Autodesk Inventor part; units mm, degrees
(part 2 of 6)
  line L607 (-11.5427, -57.3701) -> (-11.3963, -57.3701) construction
  spline S77 degree 2 poles (-11.3963, -57.3701) (-11.2792, -57.3701) (-11.0841, -57.5457) (-11.0841, -57.6677) knots 0 0 0 1 2 2 2
  line L608 (-11.3963, -57.3701) -> (-11.2792, -57.3701) construction
  line L609 (-11.2792, -57.3701) -> (-11.0841, -57.5457) construction
  line L610 (-11.0841, -57.5457) -> (-11.0841, -57.6677) construction
  spline S78 degree 2 poles (-11.0841, -57.6677) (-11.0841, -57.7506) (-11.1378, -57.8336) knots 0 0 0 1 1 1
  line L611 (-11.0841, -57.6677) -> (-11.0841, -57.7506) construction
  line L612 (-11.0841, -57.7506) -> (-11.1378, -57.8336) construction
  spline S79 degree 2 poles (-11.1378, -61.0047) (-11.0841, -61.0876) (-11.0841, -61.1705) knots 0 0 0 1 1 1
  line L613 (-11.1378, -61.0047) -> (-11.0841, -61.0876) construction
  line L614 (-11.0841, -61.0876) -> (-11.0841, -61.1705) construction
  spline S80 degree 2 poles (-11.0841, -61.1705) (-11.0841, -61.2925) (-11.2792, -61.4681) (-11.3963, -61.4681) knots 0 0 0 1 2 2 2
  line L615 (-11.0841, -61.1705) -> (-11.0841, -61.2925) construction
  line L616 (-11.0841, -61.2925) -> (-11.2792, -61.4681) construction
  line L617 (-11.2792, -61.4681) -> (-11.3963, -61.4681) construction
  spline S81 degree 2 poles (-21.1899, -61.1305) (-21.2987, -61.4569) (-21.5482, -61.4569) knots 0 0 0 1 1 1
  line L618 (-21.1899, -61.1305) -> (-21.2987, -61.4569) construction
  line L619 (-21.2987, -61.4569) -> (-21.5482, -61.4569) construction
  spline S82 degree 2 poles (-21.5482, -61.4569) (-21.8041, -61.4569) (-21.9065, -61.1305) knots 0 0 0 1 1 1
  line L620 (-21.5482, -61.4569) -> (-21.8041, -61.4569) construction
  line L621 (-21.8041, -61.4569) -> (-21.9065, -61.1305) construction
  line L622 (-21.9065, -61.1305) -> (-24.2098, -54.3101)
  spline S83 degree 2 poles (-24.2098, -54.3101) (-24.229, -54.2397) (-24.229, -54.1693) knots 0 0 0 1 1 1
  line L623 (-24.2098, -54.3101) -> (-24.229, -54.2397) construction
  line L624 (-24.229, -54.2397) -> (-24.229, -54.1693) construction
  spline S84 degree 2 poles (-24.229, -54.1693) (-24.229, -53.8046) (-23.8323, -53.8046) knots 0 0 0 1 1 1
  line L625 (-24.229, -54.1693) -> (-24.229, -53.8046) construction
  line L626 (-24.229, -53.8046) -> (-23.8323, -53.8046) construction
  spline S85 degree 2 poles (-23.8323, -53.8046) (-23.5764, -53.8046) (-23.4868, -54.0669) knots 0 0 0 1 1 1
  line L627 (-23.8323, -53.8046) -> (-23.5764, -53.8046) construction
  line L628 (-23.5764, -53.8046) -> (-23.4868, -54.0669) construction
  spline S86 degree 2 poles (-19.6095, -54.0669) (-19.52, -53.8046) (-19.264, -53.8046) knots 0 0 0 1 1 1
  line L629 (-19.6095, -54.0669) -> (-19.52, -53.8046) construction
  line L630 (-19.52, -53.8046) -> (-19.264, -53.8046) construction
  spline S87 degree 2 poles (-19.264, -53.8046) (-18.8673, -53.8046) (-18.8673, -54.1693) knots 0 0 0 1 1 1
  line L631 (-19.264, -53.8046) -> (-18.8673, -53.8046) construction
  line L632 (-18.8673, -53.8046) -> (-18.8673, -54.1693) construction
  spline S88 degree 2 poles (-18.8673, -54.1693) (-18.8673, -54.2397) (-18.8929, -54.3101) knots 0 0 0 1 1 1
  line L633 (-18.8673, -54.1693) -> (-18.8673, -54.2397) construction
  line L634 (-18.8673, -54.2397) -> (-18.8929, -54.3101) construction
  line L635 (-18.8929, -54.3101) -> (-21.1899, -61.1305)
  spline S89 degree 2 poles (16.563, -43.9283) (16.3391, -43.9283) (16.0871, -44.2083) (16.0871, -44.4042) knots 0 0 0 1 2 2 2
  line L636 (16.563, -43.9283) -> (16.3391, -43.9283) construction
  line L637 (16.3391, -43.9283) -> (16.0871, -44.2083) construction
  line L638 (16.0871, -44.2083) -> (16.0871, -44.4042) construction
  spline S90 degree 2 poles (16.0871, -44.4042) (16.0871, -44.6002) (16.2071, -44.7361) knots 0 0 0 1 1 1
  line L639 (16.0871, -44.4042) -> (16.0871, -44.6002) construction
  line L640 (16.0871, -44.6002) -> (16.2071, -44.7361) construction
  spline S91 degree 2 poles (16.2071, -44.7361) (16.3391, -44.8841) (16.563, -44.8841) knots 0 0 0 1 1 1
  line L641 (16.2071, -44.7361) -> (16.3391, -44.8841) construction
  line L642 (16.3391, -44.8841) -> (16.563, -44.8841) construction
  spline S92 degree 2 poles (16.0471, -46.6916) (15.9752, -46.8035) (15.8552, -46.8035) knots 0 0 0 1 1 1
  line L643 (16.0471, -46.6916) -> (15.9752, -46.8035) construction
  line L644 (15.9752, -46.8035) -> (15.8552, -46.8035) construction
  spline S93 degree 2 poles (15.8552, -46.8035) (15.7552, -46.8035) (15.6033, -46.6596) (15.6033, -46.5636) knots 0 0 0 1 2 2 2
  line L645 (15.8552, -46.8035) -> (15.7552, -46.8035) construction
  line L646 (15.7552, -46.8035) -> (15.6033, -46.6596) construction
  line L647 (15.6033, -46.6596) -> (15.6033, -46.5636) construction
  spline S94 degree 2 poles (15.6033, -46.5636) (15.6033, -46.4916) (15.6473, -46.4276) knots 0 0 0 1 1 1
  line L648 (15.6033, -46.5636) -> (15.6033, -46.4916) construction
  line L649 (15.6033, -46.4916) -> (15.6473, -46.4276) construction
  line L650 (15.6473, -46.4276) -> (16.3671, -45.3479)
  spline S95 degree 2 poles (16.3671, -45.3479) (16.0072, -45.288) (15.7952, -45.004) knots 0 0 0 1 1 1
  line L651 (16.3671, -45.3479) -> (16.0072, -45.288) construction
  line L652 (16.0072, -45.288) -> (15.7952, -45.004) construction
  spline S96 degree 2 poles (15.7952, -45.004) (15.6073, -44.7481) (15.6073, -44.4042) knots 0 0 0 1 1 1
  line L653 (15.7952, -45.004) -> (15.6073, -44.7481) construction
  line L654 (15.6073, -44.7481) -> (15.6073, -44.4042) construction
  spline S97 degree 2 poles (15.6073, -44.4042) (15.6073, -44.0163) (15.8472, -43.7484) knots 0 0 0 1 1 1
  line L655 (15.6073, -44.4042) -> (15.6073, -44.0163) construction
  line L656 (15.6073, -44.0163) -> (15.8472, -43.7484) construction
  spline S98 degree 2 poles (15.8472, -43.7484) (16.1111, -43.4485) (16.563, -43.4485) knots 0 0 0 1 1 1
  line L657 (15.8472, -43.7484) -> (16.1111, -43.4485) construction
  line L658 (16.1111, -43.4485) -> (16.563, -43.4485) construction
  line L659 (16.563, -43.4485) -> (17.7587, -43.4485)
  spline S99 degree 2 poles (17.7587, -43.4485) (17.9986, -43.4485) (17.9986, -43.6884) knots 0 0 0 1 1 1
  line L660 (17.7587, -43.4485) -> (17.9986, -43.4485) construction
  line L661 (17.9986, -43.4485) -> (17.9986, -43.6884) construction
  line L662 (17.9986, -43.6884) -> (17.9986, -46.5596)
  spline S100 degree 2 poles (17.9986, -46.5596) (17.9986, -46.7995) (17.7587, -46.7995) knots 0 0 0 1 1 1
  line L663 (17.9986, -46.5596) -> (17.9986, -46.7995) construction
  line L664 (17.9986, -46.7995) -> (17.7587, -46.7995) construction
  spline S101 degree 2 poles (17.7587, -46.7995) (17.5187, -46.7995) (17.5187, -46.5596) knots 0 0 0 1 1 1
  line L665 (17.7587, -46.7995) -> (17.5187, -46.7995) construction
  line L666 (17.5187, -46.7995) -> (17.5187, -46.5596) construction
  spline S102 degree 2 poles (13.6918, -46.3197) (13.8878, -46.3197) (14.1677, -46.0357) (14.1677, -45.8398) knots 0 0 0 1 2 2 2
  line L667 (13.6918, -46.3197) -> (13.8878, -46.3197) construction
  line L668 (13.8878, -46.3197) -> (14.1677, -46.0357) construction
  line L669 (14.1677, -46.0357) -> (14.1677, -45.8398) construction
  spline S103 degree 2 poles (13.2119, -43.9283) (13.016, -43.9283) (12.7361, -44.2123) (12.7361, -44.4082) knots 0 0 0 1 2 2 2
  line L670 (13.2119, -43.9283) -> (13.016, -43.9283) construction
  line L671 (13.016, -43.9283) -> (12.7361, -44.2123) construction
  line L672 (12.7361, -44.2123) -> (12.7361, -44.4082) construction
  line L673 (12.7361, -44.4082) -> (12.7361, -45.8398)
  spline S104 degree 2 poles (12.7361, -45.8398) (12.7361, -46.0357) (13.016, -46.3197) (13.2119, -46.3197) knots 0 0 0 1 2 2 2
  line L674 (12.7361, -45.8398) -> (12.7361, -46.0357) construction
  line L675 (12.7361, -46.0357) -> (13.016, -46.3197) construction
  line L676 (13.016, -46.3197) -> (13.2119, -46.3197) construction
  line L677 (13.2119, -46.3197) -> (13.6918, -46.3197)
  line L678 (13.6918, -46.7995) -> (13.2119, -46.7995)
  spline S105 degree 2 poles (13.2119, -46.7995) (12.8201, -46.7995) (12.2562, -46.2397) (12.2562, -45.8438) knots 0 0 0 1 2 2 2
  line L679 (13.2119, -46.7995) -> (12.8201, -46.7995) construction
  line L680 (12.8201, -46.7995) -> (12.2562, -46.2397) construction
  line L681 (12.2562, -46.2397) -> (12.2562, -45.8438) construction
  line L682 (12.2562, -45.8438) -> (12.2562, -44.4042)
  spline S106 degree 2 poles (12.2562, -44.4042) (12.2562, -44.0083) (12.8201, -43.4485) (13.2119, -43.4485) knots 0 0 0 1 2 2 2
  line L683 (12.2562, -44.4042) -> (12.2562, -44.0083) construction
  line L684 (12.2562, -44.0083) -> (12.8201, -43.4485) construction
  line L685 (12.8201, -43.4485) -> (13.2119, -43.4485) construction
  line L686 (13.2119, -43.4485) -> (14.4076, -43.4485)
  spline S107 degree 2 poles (14.4076, -43.4485) (14.6475, -43.4485) (14.6475, -43.6884) knots 0 0 0 1 1 1
  line L687 (14.4076, -43.4485) -> (14.6475, -43.4485) construction
  line L688 (14.6475, -43.4485) -> (14.6475, -43.6884) construction
  line L689 (14.6475, -43.6884) -> (14.6475, -45.8358)
  spline S108 degree 2 poles (14.6475, -45.8358) (14.6475, -46.1957) (14.9834, -46.3397) knots 0 0 0 1 1 1
  line L690 (14.6475, -45.8358) -> (14.6475, -46.1957) construction
  line L691 (14.6475, -46.1957) -> (14.9834, -46.3397) construction
  spline S109 degree 2 poles (14.9834, -46.3397) (15.1314, -46.3996) (15.1314, -46.5516) knots 0 0 0 1 1 1
  line L692 (14.9834, -46.3397) -> (15.1314, -46.3996) construction
  line L693 (15.1314, -46.3996) -> (15.1314, -46.5516) construction
  spline S110 degree 2 poles (15.1314, -46.5516) (15.1314, -46.6516) (14.9954, -46.8035) (14.8955, -46.8035) knots 0 0 0 1 2 2 2
  line L694 (15.1314, -46.5516) -> (15.1314, -46.6516) construction
  line L695 (15.1314, -46.6516) -> (14.9954, -46.8035) construction
  line L696 (14.9954, -46.8035) -> (14.8955, -46.8035) construction
  spline S111 degree 2 poles (14.8955, -46.8035) (14.8435, -46.8035) (14.7915, -46.7795) knots 0 0 0 1 1 1
  line L697 (14.8955, -46.8035) -> (14.8435, -46.8035) construction
  line L698 (14.8435, -46.8035) -> (14.7915, -46.7795) construction
  spline S112 degree 2 poles (14.7915, -46.7795) (14.5516, -46.6756) (14.4036, -46.4836) knots 0 0 0 1 1 1
  line L699 (14.7915, -46.7795) -> (14.5516, -46.6756) construction
  line L700 (14.5516, -46.6756) -> (14.4036, -46.4836) construction
  spline S113 degree 2 poles (14.4036, -46.4836) (14.1157, -46.7995) (13.6918, -46.7995) knots 0 0 0 1 1 1
  line L701 (14.4036, -46.4836) -> (14.1157, -46.7995) construction
  line L702 (14.1157, -46.7995) -> (13.6918, -46.7995) construction
  spline S114 degree 2 poles (-0.9121, -46.7995) (-1.152, -46.7995) (-1.152, -46.5596) knots 0 0 0 1 1 1
  line L703 (-0.9121, -46.7995) -> (-1.152, -46.7995) construction
  line L704 (-1.152, -46.7995) -> (-1.152, -46.5596) construction
  spline S115 degree 2 poles (-2.5996, -46.6356) (-2.6516, -46.7995) (-2.8115, -46.7995) knots 0 0 0 1 1 1
  line L705 (-2.5996, -46.6356) -> (-2.6516, -46.7995) construction
  line L706 (-2.6516, -46.7995) -> (-2.8115, -46.7995) construction
  spline S116 degree 2 poles (-2.8115, -46.7995) (-3.0635, -46.7995) (-3.0635, -46.5716) knots 0 0 0 1 1 1
  line L707 (-2.8115, -46.7995) -> (-3.0635, -46.7995) construction
  line L708 (-3.0635, -46.7995) -> (-3.0635, -46.5716) construction
  spline S117 degree 2 poles (-3.0635, -46.5716) (-3.0635, -46.5276) (-3.0475, -46.4836) knots 0 0 0 1 1 1
  line L709 (-3.0635, -46.5716) -> (-3.0635, -46.5276) construction
  line L710 (-3.0635, -46.5276) -> (-3.0475, -46.4836) construction
  line L711 (-3.0475, -46.4836) -> (-2.0997, -43.6124)
  spline S118 degree 2 poles (-2.0997, -43.6124) (-2.0478, -43.4485) (-1.8758, -43.4485) knots 0 0 0 1 1 1
  line L712 (-2.0997, -43.6124) -> (-2.0478, -43.4485) construction
  line L713 (-2.0478, -43.4485) -> (-1.8758, -43.4485) construction
  line L714 (-1.8758, -43.4485) -> (-0.9121, -43.4485)
  spline S119 degree 2 poles (-0.9121, -43.4485) (-0.6721, -43.4485) (-0.6721, -43.6884) knots 0 0 0 1 1 1
  line L715 (-0.9121, -43.4485) -> (-0.6721, -43.4485) construction
  line L716 (-0.6721, -43.4485) -> (-0.6721, -43.6884) construction
  line L717 (-0.6721, -43.6884) -> (-0.6721, -46.5596)
  spline S120 degree 2 poles (-0.6721, -46.5596) (-0.6721, -46.7995) (-0.9121, -46.7995) knots 0 0 0 1 1 1
  line L718 (-0.6721, -46.5596) -> (-0.6721, -46.7995) construction
  line L719 (-0.6721, -46.7995) -> (-0.9121, -46.7995) construction
  spline S121 degree 2 poles (-14.3163, -46.7995) (-14.5562, -46.7995) (-14.5562, -46.5596) knots 0 0 0 1 1 1
  line L720 (-14.3163, -46.7995) -> (-14.5562, -46.7995) construction
  line L721 (-14.5562, -46.7995) -> (-14.5562, -46.5596) construction
  line L722 (-14.5562, -46.5596) -> (-14.5562, -44.4082)
  spline S122 degree 2 poles (-14.5562, -44.4082) (-14.5562, -44.2123) (-14.8362, -43.9283) (-15.0321, -43.9283) knots 0 0 0 1 2 2 2
  line L723 (-14.5562, -44.4082) -> (-14.5562, -44.2123) construction
  line L724 (-14.5562, -44.2123) -> (-14.8362, -43.9283) construction
  line L725 (-14.8362, -43.9283) -> (-15.0321, -43.9283) construction
  spline S123 degree 2 poles (-15.9878, -46.5596) (-15.9878, -46.7995) (-16.2278, -46.7995) knots 0 0 0 1 1 1
  line L726 (-15.9878, -46.5596) -> (-15.9878, -46.7995) construction
  line L727 (-15.9878, -46.7995) -> (-16.2278, -46.7995) construction
  spline S124 degree 2 poles (-16.2278, -46.7995) (-16.4677, -46.7995) (-16.4677, -46.5596) knots 0 0 0 1 1 1
  line L728 (-16.2278, -46.7995) -> (-16.4677, -46.7995) construction
  line L729 (-16.4677, -46.7995) -> (-16.4677, -46.5596) construction
  line L730 (-16.4677, -46.5596) -> (-16.4677, -43.6884)
  spline S125 degree 2 poles (-16.4677, -43.6884) (-16.4677, -43.4485) (-16.2278, -43.4485) knots 0 0 0 1 1 1
  line L731 (-16.4677, -43.6884) -> (-16.4677, -43.4485) construction
  line L732 (-16.4677, -43.4485) -> (-16.2278, -43.4485) construction
  line L733 (-16.2278, -43.4485) -> (-15.0321, -43.4485)
  spline S126 degree 2 poles (-15.0321, -43.4485) (-14.6362, -43.4485) (-14.0764, -44.0083) (-14.0764, -44.4042) knots 0 0 0 1 2 2 2
  line L734 (-15.0321, -43.4485) -> (-14.6362, -43.4485) construction
  line L735 (-14.6362, -43.4485) -> (-14.0764, -44.0083) construction
  line L736 (-14.0764, -44.0083) -> (-14.0764, -44.4042) construction
  line L737 (-14.0764, -44.4042) -> (-14.0764, -46.5596)
  spline S127 degree 2 poles (-14.0764, -46.5596) (-14.0764, -46.7995) (-14.3163, -46.7995) knots 0 0 0 1 1 1
  line L738 (-14.0764, -46.5596) -> (-14.0764, -46.7995) construction
  line L739 (-14.0764, -46.7995) -> (-14.3163, -46.7995) construction
  spline S128 degree 2 poles (-18.3832, -46.3197) (-18.1872, -46.3197) (-17.9073, -46.0357) (-17.9073, -45.8398) knots 0 0 0 1 2 2 2
  line L740 (-18.3832, -46.3197) -> (-18.1872, -46.3197) construction
  line L741 (-18.1872, -46.3197) -> (-17.9073, -46.0357) construction
  line L742 (-17.9073, -46.0357) -> (-17.9073, -45.8398) construction
  spline S129 degree 2 poles (-18.863, -43.9283) (-19.059, -43.9283) (-19.3389, -44.2123) (-19.3389, -44.4082) knots 0 0 0 1 2 2 2
  line L743 (-18.863, -43.9283) -> (-19.059, -43.9283) construction
  line L744 (-19.059, -43.9283) -> (-19.3389, -44.2123) construction
  line L745 (-19.3389, -44.2123) -> (-19.3389, -44.4082) construction
  line L746 (-19.3389, -44.4082) -> (-19.3389, -45.8398)
  spline S130 degree 2 poles (-19.3389, -45.8398) (-19.3389, -46.0357) (-19.059, -46.3197) (-18.863, -46.3197) knots 0 0 0 1 2 2 2
  line L747 (-19.3389, -45.8398) -> (-19.3389, -46.0357) construction
  line L748 (-19.3389, -46.0357) -> (-19.059, -46.3197) construction
  line L749 (-19.059, -46.3197) -> (-18.863, -46.3197) construction
  line L750 (-18.863, -46.3197) -> (-18.3832, -46.3197)
  line L751 (-18.3832, -46.7995) -> (-18.863, -46.7995)
  spline S131 degree 2 poles (-18.863, -46.7995) (-19.2549, -46.7995) (-19.8188, -46.2397) (-19.8188, -45.8438) knots 0 0 0 1 2 2 2
  line L752 (-18.863, -46.7995) -> (-19.2549, -46.7995) construction
  line L753 (-19.2549, -46.7995) -> (-19.8188, -46.2397) construction
  line L754 (-19.8188, -46.2397) -> (-19.8188, -45.8438) construction
  line L755 (-19.8188, -45.8438) -> (-19.8188, -44.4042)
  spline S132 degree 2 poles (-19.8188, -44.4042) (-19.8188, -44.0083) (-19.2549, -43.4485) (-18.863, -43.4485) knots 0 0 0 1 2 2 2
  line L756 (-19.8188, -44.4042) -> (-19.8188, -44.0083) construction
  line L757 (-19.8188, -44.0083) -> (-19.2549, -43.4485) construction
  line L758 (-19.2549, -43.4485) -> (-18.863, -43.4485) construction
  line L759 (-18.863, -43.4485) -> (-17.6674, -43.4485)
  spline S133 degree 2 poles (-17.6674, -43.4485) (-17.4274, -43.4485) (-17.4274, -43.6884) knots 0 0 0 1 1 1
  line L760 (-17.6674, -43.4485) -> (-17.4274, -43.4485) construction
  line L761 (-17.4274, -43.4485) -> (-17.4274, -43.6884) construction
  line L762 (-17.4274, -43.6884) -> (-17.4274, -45.8358)
  spline S134 degree 2 poles (-17.4274, -45.8358) (-17.4274, -46.1957) (-17.0915, -46.3397) knots 0 0 0 1 1 1
  line L763 (-17.4274, -45.8358) -> (-17.4274, -46.1957) construction
  line L764 (-17.4274, -46.1957) -> (-17.0915, -46.3397) construction
  spline S135 degree 2 poles (-17.0915, -46.3397) (-16.9436, -46.3996) (-16.9436, -46.5516) knots 0 0 0 1 1 1
  line L765 (-17.0915, -46.3397) -> (-16.9436, -46.3996) construction
  line L766 (-16.9436, -46.3996) -> (-16.9436, -46.5516) construction
  spline S136 degree 2 poles (-16.9436, -46.5516) (-16.9436, -46.6516) (-17.0795, -46.8035) (-17.1795, -46.8035) knots 0 0 0 1 2 2 2
  line L767 (-16.9436, -46.5516) -> (-16.9436, -46.6516) construction
  line L768 (-16.9436, -46.6516) -> (-17.0795, -46.8035) construction
  line L769 (-17.0795, -46.8035) -> (-17.1795, -46.8035) construction
  spline S137 degree 2 poles (-17.1795, -46.8035) (-17.2315, -46.8035) (-17.2835, -46.7795) knots 0 0 0 1 1 1
  line L770 (-17.1795, -46.8035) -> (-17.2315, -46.8035) construction
  line L771 (-17.2315, -46.8035) -> (-17.2835, -46.7795) construction
  spline S138 degree 2 poles (-17.2835, -46.7795) (-17.5234, -46.6756) (-17.6714, -46.4836) knots 0 0 0 1 1 1
  line L772 (-17.2835, -46.7795) -> (-17.5234, -46.6756) construction
  line L773 (-17.5234, -46.6756) -> (-17.6714, -46.4836) construction
  spline S139 degree 2 poles (-17.6714, -46.4836) (-17.9593, -46.7995) (-18.3832, -46.7995) knots 0 0 0 1 1 1
  line L774 (-17.6714, -46.4836) -> (-17.9593, -46.7995) construction
  line L775 (-17.9593, -46.7995) -> (-18.3832, -46.7995) construction
  spline S140 degree 2 poles (13.8884, -35.5379) (13.4965, -35.5379) (12.9287, -34.9781) (12.9287, -34.5822) knots 0 0 0 1 2 2 2
  line L776 (13.8884, -35.5379) -> (13.4965, -35.5379) construction
  line L777 (13.4965, -35.5379) -> (12.9287, -34.9781) construction
  line L778 (12.9287, -34.9781) -> (12.9287, -34.5822) construction
  line L779 (12.9287, -34.5822) -> (12.9287, -33.1426)
  spline S141 degree 2 poles (12.9287, -33.1426) (12.9287, -32.7467) (13.4965, -32.1868) (13.8884, -32.1868) knots 0 0 0 1 2 2 2
  line L780 (12.9287, -33.1426) -> (12.9287, -32.7467) construction
  line L781 (12.9287, -32.7467) -> (13.4965, -32.1868) construction
  line L782 (13.4965, -32.1868) -> (13.8884, -32.1868) construction
  line L783 (13.8884, -32.1868) -> (14.6042, -32.1868)
  spline S142 degree 2 poles (14.6042, -32.1868) (14.8441, -32.1868) (14.8441, -32.4268) knots 0 0 0 1 1 1
  line L784 (14.6042, -32.1868) -> (14.8441, -32.1868) construction
  line L785 (14.8441, -32.1868) -> (14.8441, -32.4268) construction
  spline S143 degree 2 poles (14.8441, -32.4268) (14.8441, -32.6667) (14.6042, -32.6667) knots 0 0 0 1 1 1
  line L786 (14.8441, -32.4268) -> (14.8441, -32.6667) construction
  line L787 (14.8441, -32.6667) -> (14.6042, -32.6667) construction
  line L788 (14.6042, -32.6667) -> (13.8884, -32.6667)
  spline S144 degree 2 poles (13.8884, -32.6667) (13.6925, -32.6667) (13.4085, -32.9506) (13.4085, -33.1466) knots 0 0 0 1 2 2 2
  line L789 (13.8884, -32.6667) -> (13.6925, -32.6667) construction
  line L790 (13.6925, -32.6667) -> (13.4085, -32.9506) construction
  line L791 (13.4085, -32.9506) -> (13.4085, -33.1466) construction
  line L792 (13.4085, -33.1466) -> (13.4085, -34.5782)
  spline S145 degree 2 poles (13.4085, -34.5782) (13.4085, -34.7741) (13.6925, -35.058) (13.8884, -35.058) knots 0 0 0 1 2 2 2
  line L793 (13.4085, -34.5782) -> (13.4085, -34.7741) construction
  line L794 (13.4085, -34.7741) -> (13.6925, -35.058) construction
  line L795 (13.6925, -35.058) -> (13.8884, -35.058) construction
  line L796 (13.8884, -35.058) -> (14.6042, -35.058)
  spline S146 degree 2 poles (14.6042, -35.058) (14.8441, -35.058) (14.8441, -35.298) knots 0 0 0 1 1 1
  line L797 (14.6042, -35.058) -> (14.8441, -35.058) construction
  line L798 (14.8441, -35.058) -> (14.8441, -35.298) construction
  spline S147 degree 2 poles (14.8441, -35.298) (14.8441, -35.5379) (14.6042, -35.5379) knots 0 0 0 1 1 1
  line L799 (14.8441, -35.298) -> (14.8441, -35.5379) construction
  line L800 (14.8441, -35.5379) -> (14.6042, -35.5379) construction
  line L801 (14.6042, -35.5379) -> (13.8884, -35.5379)
  spline S148 degree 2 poles (25.8131, -22.0572) (26.053, -22.0572) (26.053, -22.2971) knots 0 0 0 1 1 1
  line L802 (25.8131, -22.0572) -> (26.053, -22.0572) construction
  line L803 (26.053, -22.0572) -> (26.053, -22.2971) construction
  spline S149 degree 2 poles (26.053, -22.2971) (26.053, -22.5371) (25.8131, -22.5371) knots 0 0 0 1 1 1
  line L804 (26.053, -22.2971) -> (26.053, -22.5371) construction
  line L805 (26.053, -22.5371) -> (25.8131, -22.5371) construction
  spline S150 degree 2 poles (25.8131, -22.5371) (25.5731, -22.5371) (25.5731, -22.2971) knots 0 0 0 1 1 1
  line L806 (25.8131, -22.5371) -> (25.5731, -22.5371) construction
  line L807 (25.5731, -22.5371) -> (25.5731, -22.2971) construction
  spline S151 degree 2 poles (25.5731, -22.2971) (25.5731, -22.0572) (25.8131, -22.0572) knots 0 0 0 1 1 1
  line L808 (25.5731, -22.2971) -> (25.5731, -22.0572) construction
  line L809 (25.5731, -22.0572) -> (25.8131, -22.0572) construction
  spline S152 degree 2 poles (23.6577, -22.0572) (23.8536, -22.0572) (24.1335, -21.7733) (24.1335, -21.5773) knots 0 0 0 1 2 2 2
  line L810 (23.6577, -22.0572) -> (23.8536, -22.0572) construction
  line L811 (23.8536, -22.0572) -> (24.1335, -21.7733) construction
  line L812 (24.1335, -21.7733) -> (24.1335, -21.5773) construction
  line L813 (24.1335, -21.5773) -> (24.1335, -20.1458)
  spline S153 degree 2 poles (24.1335, -20.1458) (24.1335, -19.9498) (23.8536, -19.6659) (23.6577, -19.6659) knots 0 0 0 1 2 2 2
  line L814 (24.1335, -20.1458) -> (24.1335, -19.9498) construction
  line L815 (24.1335, -19.9498) -> (23.8536, -19.6659) construction
  line L816 (23.8536, -19.6659) -> (23.6577, -19.6659) construction
  spline S154 degree 2 poles (22.7019, -23.7327) (22.7019, -23.9727) (22.462, -23.9727) knots 0 0 0 1 1 1
  line L817 (22.7019, -23.7327) -> (22.7019, -23.9727) construction
  line L818 (22.7019, -23.9727) -> (22.462, -23.9727) construction
  spline S155 degree 2 poles (22.462, -23.9727) (22.2221, -23.9727) (22.2221, -23.7327) knots 0 0 0 1 1 1
  line L819 (22.462, -23.9727) -> (22.2221, -23.9727) construction
  line L820 (22.2221, -23.9727) -> (22.2221, -23.7327) construction
  line L821 (22.2221, -23.7327) -> (22.2221, -19.426)
  spline S156 degree 2 poles (22.2221, -19.426) (22.2221, -19.186) (22.462, -19.186) knots 0 0 0 1 1 1
  line L822 (22.2221, -19.426) -> (22.2221, -19.186) construction
  line L823 (22.2221, -19.186) -> (22.462, -19.186) construction
  line L824 (22.462, -19.186) -> (23.6577, -19.186)
  spline S157 degree 2 poles (23.6577, -19.186) (24.0535, -19.186) (24.6134, -19.7459) (24.6134, -20.1418) knots 0 0 0 1 2 2 2
  line L825 (23.6577, -19.186) -> (24.0535, -19.186) construction
  line L826 (24.0535, -19.186) -> (24.6134, -19.7459) construction
  line L827 (24.6134, -19.7459) -> (24.6134, -20.1418) construction
  line L828 (24.6134, -20.1418) -> (24.6134, -21.5813)
  spline S158 degree 2 poles (24.6134, -21.5813) (24.6134, -21.9772) (24.0535, -22.5371) (23.6577, -22.5371) knots 0 0 0 1 2 2 2
  line L829 (24.6134, -21.5813) -> (24.6134, -21.9772) construction
  line L830 (24.6134, -21.9772) -> (24.0535, -22.5371) construction
  line L831 (24.0535, -22.5371) -> (23.6577, -22.5371) construction
  spline S159 degree 2 poles (20.7825, -20.1418) (20.7825, -19.9458) (20.5025, -19.6659) (20.3066, -19.6659) knots 0 0 0 1 2 2 2
  line L832 (20.7825, -20.1418) -> (20.7825, -19.9458) construction
  line L833 (20.7825, -19.9458) -> (20.5025, -19.6659) construction
  line L834 (20.5025, -19.6659) -> (20.3066, -19.6659) construction
  line L835 (20.3066, -19.6659) -> (19.8267, -19.6659)
  spline S160 degree 2 poles (19.8267, -19.6659) (19.6308, -19.6659) (19.3509, -19.9458) (19.3509, -20.1418) knots 0 0 0 1 2 2 2
  line L836 (19.8267, -19.6659) -> (19.6308, -19.6659) construction
  line L837 (19.6308, -19.6659) -> (19.3509, -19.9458) construction
  line L838 (19.3509, -19.9458) -> (19.3509, -20.1418) construction
  spline S161 degree 2 poles (19.3509, -21.5773) (19.3509, -21.7733) (19.6348, -22.0572) (19.8307, -22.0572) knots 0 0 0 1 2 2 2
  line L839 (19.3509, -21.5773) -> (19.3509, -21.7733) construction
  line L840 (19.3509, -21.7733) -> (19.6348, -22.0572) construction
  line L841 (19.6348, -22.0572) -> (19.8307, -22.0572) construction
  line L842 (19.8307, -22.0572) -> (21.0224, -22.0572)
  spline S162 degree 2 poles (21.0224, -22.0572) (21.2623, -22.0572) (21.2623, -22.2971) knots 0 0 0 1 1 1
  line L843 (21.0224, -22.0572) -> (21.2623, -22.0572) construction
  line L844 (21.2623, -22.0572) -> (21.2623, -22.2971) construction
  spline S163 degree 2 poles (21.2623, -22.2971) (21.2623, -22.5371) (21.0224, -22.5371) knots 0 0 0 1 1 1
  line L845 (21.2623, -22.2971) -> (21.2623, -22.5371) construction
  line L846 (21.2623, -22.5371) -> (21.0224, -22.5371) construction
  line L847 (21.0224, -22.5371) -> (19.8267, -22.5371)
  spline S164 degree 2 poles (19.8267, -22.5371) (19.4309, -22.5371) (18.871, -21.9772) (18.871, -21.5813) knots 0 0 0 1 2 2 2
  line L848 (19.8267, -22.5371) -> (19.4309, -22.5371) construction
  line L849 (19.4309, -22.5371) -> (18.871, -21.9772) construction
  line L850 (18.871, -21.9772) -> (18.871, -21.5813) construction
  line L851 (18.871, -21.5813) -> (18.871, -20.1418)
  spline S165 degree 2 poles (18.871, -20.1418) (18.871, -19.7459) (19.4309, -19.186) (19.8267, -19.186) knots 0 0 0 1 2 2 2
  line L852 (18.871, -20.1418) -> (18.871, -19.7459) construction
  line L853 (18.871, -19.7459) -> (19.4309, -19.186) construction
  line L854 (19.4309, -19.186) -> (19.8267, -19.186) construction
  line L855 (19.8267, -19.186) -> (20.3066, -19.186)
  spline S166 degree 2 poles (20.3066, -19.186) (20.7025, -19.186) (21.2623, -19.7459) (21.2623, -20.1418) knots 0 0 0 1 2 2 2
  line L856 (20.3066, -19.186) -> (20.7025, -19.186) construction
  line L857 (20.7025, -19.186) -> (21.2623, -19.7459) construction
  line L858 (21.2623, -19.7459) -> (21.2623, -20.1418) construction
  line L859 (21.2623, -20.1418) -> (21.2623, -20.8615)
  spline S167 degree 2 poles (21.2623, -20.8615) (21.2623, -21.1015) (21.0224, -21.1015) knots 0 0 0 1 1 1
  line L860 (21.2623, -20.8615) -> (21.2623, -21.1015) construction
  line L861 (21.2623, -21.1015) -> (21.0224, -21.1015) construction
  spline S168 degree 2 poles (12.8847, -21.1015) (12.6448, -21.1015) (12.6448, -20.8615) knots 0 0 0 1 1 1
  line L862 (12.8847, -21.1015) -> (12.6448, -21.1015) construction
  line L863 (12.6448, -21.1015) -> (12.6448, -20.8615) construction
  spline S169 degree 2 poles (12.6448, -20.8615) (12.6448, -20.6216) (12.8847, -20.6216) knots 0 0 0 1 1 1
  line L864 (12.6448, -20.8615) -> (12.6448, -20.6216) construction
  line L865 (12.6448, -20.6216) -> (12.8847, -20.6216) construction
  line L866 (12.8847, -20.6216) -> (13.1246, -20.6216)
  spline S170 degree 2 poles (13.1246, -20.6216) (13.3486, -20.6216) (13.4805, -20.4737) knots 0 0 0 1 1 1
  line L867 (13.1246, -20.6216) -> (13.3486, -20.6216) construction
  line L868 (13.3486, -20.6216) -> (13.4805, -20.4737) construction
  spline S171 degree 2 poles (13.4805, -20.4737) (13.6005, -20.3377) (13.6005, -20.1418) knots 0 0 0 1 1 1
  line L869 (13.4805, -20.4737) -> (13.6005, -20.3377) construction
  line L870 (13.6005, -20.3377) -> (13.6005, -20.1418) construction
  spline S172 degree 2 poles (13.6005, -20.1418) (13.6005, -19.9458) (13.4805, -19.8138) knots 0 0 0 1 1 1
  line L871 (13.6005, -20.1418) -> (13.6005, -19.9458) construction
  line L872 (13.6005, -19.9458) -> (13.4805, -19.8138) construction
  spline S173 degree 2 poles (13.4805, -19.8138) (13.3486, -19.6659) (13.1206, -19.6659) knots 0 0 0 1 1 1
  line L873 (13.4805, -19.8138) -> (13.3486, -19.6659) construction
  line L874 (13.3486, -19.6659) -> (13.1206, -19.6659) construction
  line L875 (13.1206, -19.6659) -> (12.8807, -19.6659)
  spline S174 degree 2 poles (12.8807, -19.6659) (12.5568, -19.6659) (12.3089, -19.8578) knots 0 0 0 1 1 1
  line L876 (12.8807, -19.6659) -> (12.5568, -19.6659) construction
  line L877 (12.5568, -19.6659) -> (12.3089, -19.8578) construction
  spline S175 degree 2 poles (12.3089, -19.8578) (12.2369, -19.9098) (12.1609, -19.9098) knots 0 0 0 1 1 1
  line L878 (12.3089, -19.8578) -> (12.2369, -19.9098) construction
  line L879 (12.2369, -19.9098) -> (12.1609, -19.9098) construction
  spline S176 degree 2 poles (12.1609, -19.9098) (12.0649, -19.9098) (11.921, -19.7619) (11.921, -19.6619) knots 0 0 0 1 2 2 2
  line L880 (12.1609, -19.9098) -> (12.0649, -19.9098) construction
  line L881 (12.0649, -19.9098) -> (11.921, -19.7619) construction
  line L882 (11.921, -19.7619) -> (11.921, -19.6619) construction
  spline S177 degree 2 poles (11.921, -19.6619) (11.921, -19.5499) (12.0209, -19.4739) knots 0 0 0 1 1 1
  line L883 (11.921, -19.6619) -> (11.921, -19.5499) construction
  line L884 (11.921, -19.5499) -> (12.0209, -19.4739) construction
  spline S178 degree 2 poles (12.0209, -19.4739) (12.3928, -19.186) (12.8807, -19.186) knots 0 0 0 1 1 1
  line L885 (12.0209, -19.4739) -> (12.3928, -19.186) construction
  line L886 (12.3928, -19.186) -> (12.8807, -19.186) construction
  line L887 (12.8807, -19.186) -> (13.1206, -19.186)
  spline S179 degree 2 poles (13.1206, -19.186) (13.5725, -19.186) (13.8404, -19.4819) knots 0 0 0 1 1 1
  line L888 (13.1206, -19.186) -> (13.5725, -19.186) construction
  line L889 (13.5725, -19.186) -> (13.8404, -19.4819) construction
  spline S180 degree 2 poles (13.8404, -19.4819) (14.0804, -19.7539) (14.0804, -20.1418) knots 0 0 0 1 1 1
  line L890 (13.8404, -19.4819) -> (14.0804, -19.7539) construction
  line L891 (14.0804, -19.7539) -> (14.0804, -20.1418) construction
  spline S181 degree 2 poles (14.0804, -20.1418) (14.0804, -20.5856) (13.7804, -20.8615) knots 0 0 0 1 1 1
  line L892 (14.0804, -20.1418) -> (14.0804, -20.5856) construction
  line L893 (14.0804, -20.5856) -> (13.7804, -20.8615) construction
  spline S182 degree 2 poles (13.7804, -20.8615) (14.0804, -21.1375) (14.0804, -21.5813) knots 0 0 0 1 1 1
  line L894 (13.7804, -20.8615) -> (14.0804, -21.1375) construction
  line L895 (14.0804, -21.1375) -> (14.0804, -21.5813) construction
  spline S183 degree 2 poles (14.0804, -21.5813) (14.0804, -21.9732) (13.8404, -22.2412) knots 0 0 0 1 1 1
  line L896 (14.0804, -21.5813) -> (14.0804, -21.9732) construction
  line L897 (14.0804, -21.9732) -> (13.8404, -22.2412) construction
  spline S184 degree 2 poles (13.8404, -22.2412) (13.5725, -22.5371) (13.1206, -22.5371) knots 0 0 0 1 1 1
  line L898 (13.8404, -22.2412) -> (13.5725, -22.5371) construction
  line L899 (13.5725, -22.5371) -> (13.1206, -22.5371) construction
  line L900 (13.1206, -22.5371) -> (12.8807, -22.5371)
  spline S185 degree 2 poles (12.8807, -22.5371) (12.3928, -22.5371) (12.0209, -22.2492) knots 0 0 0 1 1 1
  line L901 (12.8807, -22.5371) -> (12.3928, -22.5371) construction
  line L902 (12.3928, -22.5371) -> (12.0209, -22.2492) construction
  spline S186 degree 2 poles (12.0209, -22.2492) (11.921, -22.1732) (11.921, -22.0612) knots 0 0 0 1 1 1
  line L903 (12.0209, -22.2492) -> (11.921, -22.1732) construction
  line L904 (11.921, -22.1732) -> (11.921, -22.0612) construction
  spline S187 degree 2 poles (11.921, -22.0612) (11.921, -21.9612) (12.0649, -21.8133) (12.1609, -21.8133) knots 0 0 0 1 2 2 2
  line L905 (11.921, -22.0612) -> (11.921, -21.9612) construction
  line L906 (11.921, -21.9612) -> (12.0649, -21.8133) construction
  line L907 (12.0649, -21.8133) -> (12.1609, -21.8133) construction
  spline S188 degree 2 poles (12.1609, -21.8133) (12.2369, -21.8133) (12.3089, -21.8653) knots 0 0 0 1 1 1
  line L908 (12.1609, -21.8133) -> (12.2369, -21.8133) construction
  line L909 (12.2369, -21.8133) -> (12.3089, -21.8653) construction
  spline S189 degree 2 poles (12.3089, -21.8653) (12.5568, -22.0572) (12.8807, -22.0572) knots 0 0 0 1 1 1
  line L910 (12.3089, -21.8653) -> (12.5568, -22.0572) construction
  line L911 (12.5568, -22.0572) -> (12.8807, -22.0572) construction
  line L912 (12.8807, -22.0572) -> (13.1206, -22.0572)
  spline S190 degree 2 poles (13.1206, -22.0572) (13.3486, -22.0572) (13.4805, -21.9053) knots 0 0 0 1 1 1
  line L913 (13.1206, -22.0572) -> (13.3486, -22.0572) construction
  line L914 (13.3486, -22.0572) -> (13.4805, -21.9053) construction
  spline S191 degree 2 poles (13.4805, -21.9053) (13.6005, -21.7693) (13.6005, -21.5733) knots 0 0 0 1 1 1
  line L915 (13.4805, -21.9053) -> (13.6005, -21.7693) construction
  line L916 (13.6005, -21.7693) -> (13.6005, -21.5733) construction
  spline S192 degree 2 poles (13.6005, -21.5733) (13.6005, -21.1455) (13.1846, -21.1015) knots 0 0 0 1 1 1
  line L917 (13.6005, -21.5733) -> (13.6005, -21.1455) construction
  line L918 (13.6005, -21.1455) -> (13.1846, -21.1015) construction
  line L919 (13.1846, -21.1015) -> (12.8847, -21.1015)
  spline S193 degree 2 poles (-21.2108, -37.1301) (-21.4508, -37.1301) (-21.4508, -36.8902) knots 0 0 0 1 1 1
  line L920 (-21.2108, -37.1301) -> (-21.4508, -37.1301) construction
  line L921 (-21.4508, -37.1301) -> (-21.4508, -36.8902) construction
  line L922 (-21.4508, -36.8902) -> (-21.4508, -32.5834)
  spline S194 degree 2 poles (-21.4508, -32.5834) (-21.4508, -32.3434) (-21.2108, -32.3434) knots 0 0 0 1 1 1
  line L923 (-21.4508, -32.5834) -> (-21.4508, -32.3434) construction
  line L924 (-21.4508, -32.3434) -> (-21.2108, -32.3434) construction
  spline S195 degree 2 poles (-21.2108, -32.3434) (-20.9709, -32.3434) (-20.9709, -32.5834) knots 0 0 0 1 1 1
  line L925 (-21.2108, -32.3434) -> (-20.9709, -32.3434) construction
  line L926 (-20.9709, -32.3434) -> (-20.9709, -32.5834) construction
  spline S196 degree 2 poles (-19.2954, -36.6502) (-19.0555, -36.6502) (-19.0555, -36.8902) knots 0 0 0 1 1 1
  line L927 (-19.2954, -36.6502) -> (-19.0555, -36.6502) construction
  line L928 (-19.0555, -36.6502) -> (-19.0555, -36.8902) construction
  spline S197 degree 2 poles (-19.0555, -36.8902) (-19.0555, -37.1301) (-19.2954, -37.1301) knots 0 0 0 1 1 1
  line L929 (-19.0555, -36.8902) -> (-19.0555, -37.1301) construction
  line L930 (-19.0555, -37.1301) -> (-19.2954, -37.1301) construction
  line L931 (-19.2954, -37.1301) -> (-21.2108, -37.1301)
  spline S198 degree 2 poles (-22.8323, -26.6241) (-22.8323, -26.7201) (-22.9763, -26.8721) (-23.0722, -26.8721) knots 0 0 0 1 2 2 2
  line L932 (-22.8323, -26.6241) -> (-22.8323, -26.7201) construction
  line L933 (-22.8323, -26.7201) -> (-22.9763, -26.8721) construction
  line L934 (-22.9763, -26.8721) -> (-23.0722, -26.8721) construction
  spline S199 degree 2 poles (-23.0722, -26.8721) (-23.1482, -26.8721) (-23.2162, -26.8241) knots 0 0 0 1 1 1
  line L935 (-23.0722, -26.8721) -> (-23.1482, -26.8721) construction
  line L936 (-23.1482, -26.8721) -> (-23.2162, -26.8241) construction
  spline S200 degree 2 poles (-23.2162, -26.8241) (-23.6721, -26.4962) (-24.2279, -26.4962) knots 0 0 0 1 1 1
  line L937 (-23.2162, -26.8241) -> (-23.6721, -26.4962) construction
  line L938 (-23.6721, -26.4962) -> (-24.2279, -26.4962) construction
  spline S201 degree 2 poles (-24.2279, -26.4962) (-24.5878, -26.4962) (-25.1677, -26.7961) (-25.1677, -27.084) knots 0 0 0 1 2 2 2
  line L939 (-24.2279, -26.4962) -> (-24.5878, -26.4962) construction
  line L940 (-24.5878, -26.4962) -> (-25.1677, -26.7961) construction
  line L941 (-25.1677, -26.7961) -> (-25.1677, -27.084) construction
  spline S202 degree 2 poles (-25.1677, -27.084) (-25.1677, -27.256) (-25.0317, -27.3599) knots 0 0 0 1 1 1
  line L942 (-25.1677, -27.084) -> (-25.1677, -27.256) construction
  line L943 (-25.1677, -27.256) -> (-25.0317, -27.3599) construction
  line L944 (-25.0317, -27.3599) -> (-23.2562, -28.6716)
  spline S203 degree 2 poles (-23.2562, -28.6716) (-22.7763, -29.0235) (-22.7763, -29.6553) knots 0 0 0 1 1 1
  line L945 (-23.2562, -28.6716) -> (-22.7763, -29.0235) construction
  line L946 (-22.7763, -29.0235) -> (-22.7763, -29.6553) construction
  spline S204 degree 2 poles (-22.7763, -29.6553) (-22.7763, -30.3111) (-23.784, -30.8389) (-24.2679, -30.8389) knots 0 0 0 1 2 2 2
  line L947 (-22.7763, -29.6553) -> (-22.7763, -30.3111) construction
  line L948 (-22.7763, -30.3111) -> (-23.784, -30.8389) construction
  line L949 (-23.784, -30.8389) -> (-24.2679, -30.8389) construction
  spline S205 degree 2 poles (-24.2679, -30.8389) (-24.8757, -30.8389) (-25.5355, -30.4111) knots 0 0 0 1 1 1
  line L950 (-24.2679, -30.8389) -> (-24.8757, -30.8389) construction
  line L951 (-24.8757, -30.8389) -> (-25.5355, -30.4111) construction
  spline S206 degree 2 poles (-25.5355, -30.4111) (-25.6475, -30.3391) (-25.6475, -30.2191) knots 0 0 0 1 1 1
  line L952 (-25.5355, -30.4111) -> (-25.6475, -30.3391) construction
  line L953 (-25.6475, -30.3391) -> (-25.6475, -30.2191) construction
  spline S207 degree 2 poles (-25.6475, -30.2191) (-25.6475, -30.1192) (-25.5076, -29.9672) (-25.4076, -29.9672) knots 0 0 0 1 2 2 2
  line L954 (-25.6475, -30.2191) -> (-25.6475, -30.1192) construction
  line L955 (-25.6475, -30.1192) -> (-25.5076, -29.9672) construction
  line L956 (-25.5076, -29.9672) -> (-25.4076, -29.9672) construction
  spline S208 degree 2 poles (-25.4076, -29.9672) (-25.3396, -29.9672) (-25.2796, -30.0112) knots 0 0 0 1 1 1
  line L957 (-25.4076, -29.9672) -> (-25.3396, -29.9672) construction
  line L958 (-25.3396, -29.9672) -> (-25.2796, -30.0112) construction
  spline S209 degree 2 poles (-25.2796, -30.0112) (-24.7358, -30.3591) (-24.2559, -30.3591) knots 0 0 0 1 1 1
  line L959 (-25.2796, -30.0112) -> (-24.7358, -30.3591) construction
  line L960 (-24.7358, -30.3591) -> (-24.2559, -30.3591) construction
  spline S210 degree 2 poles (-24.2559, -30.3591) (-23.888, -30.3591) (-23.5001, -30.1591) knots 0 0 0 1 1 1
  line L961 (-24.2559, -30.3591) -> (-23.888, -30.3591) construction
  line L962 (-23.888, -30.3591) -> (-23.5001, -30.1591) construction
  spline S211 degree 2 poles (-23.5001, -30.1591) (-23.2402, -30.0192) (-23.2402, -29.6633) knots 0 0 0 1 1 1
  line L963 (-23.5001, -30.1591) -> (-23.2402, -30.0192) construction
  line L964 (-23.2402, -30.0192) -> (-23.2402, -29.6633) construction
  spline S212 degree 2 poles (-23.2402, -29.6633) (-23.2402, -29.2754) (-23.5241, -29.0674) knots 0 0 0 1 1 1
  line L965 (-23.2402, -29.6633) -> (-23.2402, -29.2754) construction
  line L966 (-23.2402, -29.2754) -> (-23.5241, -29.0674) construction
  line L967 (-23.5241, -29.0674) -> (-25.2996, -27.7518)
  spline S213 degree 2 poles (-25.2996, -27.7518) (-25.6275, -27.5119) (-25.6275, -27.076) knots 0 0 0 1 1 1
  line L968 (-25.2996, -27.7518) -> (-25.6275, -27.5119) construction
  line L969 (-25.6275, -27.5119) -> (-25.6275, -27.076) construction
  spline S214 degree 2 poles (-25.6275, -27.076) (-25.6275, -26.5042) (-25.0957, -26.2242) knots 0 0 0 1 1 1
  line L970 (-25.6275, -27.076) -> (-25.6275, -26.5042) construction
  line L971 (-25.6275, -26.5042) -> (-25.0957, -26.2242) construction
  spline S215 degree 2 poles (-25.0957, -26.2242) (-24.7118, -26.0283) (-24.2279, -26.0283) knots 0 0 0 1 1 1
  line L972 (-25.0957, -26.2242) -> (-24.7118, -26.0283) construction
  line L973 (-24.7118, -26.0283) -> (-24.2279, -26.0283) construction
  spline S216 degree 2 poles (-24.2279, -26.0283) (-23.5081, -26.0283) (-22.9403, -26.4322) knots 0 0 0 1 1 1
  line L974 (-24.2279, -26.0283) -> (-23.5081, -26.0283) construction
  line L975 (-23.5081, -26.0283) -> (-22.9403, -26.4322) construction
  spline S217 degree 2 poles (-22.9403, -26.4322) (-22.8323, -26.5082) (-22.8323, -26.6241) knots 0 0 0 1 1 1
  line L976 (-22.9403, -26.4322) -> (-22.8323, -26.5082) construction
  line L977 (-22.8323, -26.5082) -> (-22.8323, -26.6241) construction
  spline S218 degree 2 poles (-7.2481, -22.1122) (-7.0242, -22.1122) (-6.8922, -21.9642) knots 0 0 0 1 1 1
  line L978 (-7.2481, -22.1122) -> (-7.0242, -22.1122) construction
  line L979 (-7.0242, -22.1122) -> (-6.8922, -21.9642) construction
  spline S219 degree 2 poles (-6.8922, -21.9642) (-6.7722, -21.8283) (-6.7722, -21.6323) knots 0 0 0 1 1 1
  line L980 (-6.8922, -21.9642) -> (-6.7722, -21.8283) construction
  line L981 (-6.7722, -21.8283) -> (-6.7722, -21.6323) construction
  spline S220 degree 2 poles (-6.7722, -21.6323) (-6.7722, -21.4364) (-6.8922, -21.3044) knots 0 0 0 1 1 1
  line L982 (-6.7722, -21.6323) -> (-6.7722, -21.4364) construction
  line L983 (-6.7722, -21.4364) -> (-6.8922, -21.3044) construction
  spline S221 degree 2 poles (-6.8922, -21.3044) (-7.0242, -21.1565) (-7.2481, -21.1565) knots 0 0 0 1 1 1
  line L984 (-6.8922, -21.3044) -> (-7.0242, -21.1565) construction
  line L985 (-7.0242, -21.1565) -> (-7.2481, -21.1565) construction
  spline S222 degree 2 poles (-7.2481, -20.6766) (-6.7922, -20.6766) (-6.5323, -20.9765) knots 0 0 0 1 1 1
  line L986 (-7.2481, -20.6766) -> (-6.7922, -20.6766) construction
  line L987 (-6.7922, -20.6766) -> (-6.5323, -20.9765) construction
  spline S223 degree 2 poles (-6.5323, -20.9765) (-6.2924, -21.2444) (-6.2924, -21.6323) knots 0 0 0 1 1 1
  line L988 (-6.5323, -20.9765) -> (-6.2924, -21.2444) construction
  line L989 (-6.2924, -21.2444) -> (-6.2924, -21.6323) construction
  spline S224 degree 2 poles (-6.2924, -21.6323) (-6.2924, -22.0202) (-6.5323, -22.2961) knots 0 0 0 1 1 1
  line L990 (-6.2924, -21.6323) -> (-6.2924, -22.0202) construction
  line L991 (-6.2924, -22.0202) -> (-6.5323, -22.2961) construction
  spline S225 degree 2 poles (-6.5323, -22.2961) (-6.7962, -22.5921) (-7.2481, -22.5921) knots 0 0 0 1 1 1
  line L992 (-6.5323, -22.2961) -> (-6.7962, -22.5921) construction
  line L993 (-6.7962, -22.5921) -> (-7.2481, -22.5921) construction
  line L994 (-7.2481, -22.5921) -> (-8.4438, -22.5921)
  spline S226 degree 2 poles (-8.4438, -22.5921) (-8.6837, -22.5921) (-8.6837, -22.3521) knots 0 0 0 1 1 1
  line L995 (-8.4438, -22.5921) -> (-8.6837, -22.5921) construction
  line L996 (-8.6837, -22.5921) -> (-8.6837, -22.3521) construction
  line L997 (-8.6837, -22.3521) -> (-8.6837, -19.4809)
  spline S227 degree 2 poles (-8.6837, -19.4809) (-8.6837, -19.241) (-8.4438, -19.241) knots 0 0 0 1 1 1
  line L998 (-8.6837, -19.4809) -> (-8.6837, -19.241) construction
  line L999 (-8.6837, -19.241) -> (-8.4438, -19.241) construction
  spline S228 degree 2 poles (-8.4438, -19.241) (-8.2038, -19.241) (-8.2038, -19.4809) knots 0 0 0 1 1 1
  line L1000 (-8.4438, -19.241) -> (-8.2038, -19.241) construction
  line L1001 (-8.2038, -19.241) -> (-8.2038, -19.4809) construction
  line L1002 (-12.7546, -22.5921) -> (-13.9502, -22.5921)
  spline S229 degree 2 poles (-13.9502, -22.5921) (-14.3421, -22.5921) (-14.906, -22.0322) (-14.906, -21.6363) knots 0 0 0 1 2 2 2
  line L1003 (-13.9502, -22.5921) -> (-14.3421, -22.5921) construction
  line L1004 (-14.3421, -22.5921) -> (-14.906, -22.0322) construction
  line L1005 (-14.906, -22.0322) -> (-14.906, -21.6363) construction
  line L1006 (-14.906, -21.6363) -> (-14.906, -19.4809)
  spline S230 degree 2 poles (-14.906, -19.4809) (-14.906, -19.241) (-14.666, -19.241) knots 0 0 0 1 1 1
  line L1007 (-14.906, -19.4809) -> (-14.906, -19.241) construction
  line L1008 (-14.906, -19.241) -> (-14.666, -19.241) construction
  spline S231 degree 2 poles (-14.666, -19.241) (-14.4261, -19.241) (-14.4261, -19.4809) knots 0 0 0 1 1 1
  line L1009 (-14.666, -19.241) -> (-14.4261, -19.241) construction
  line L1010 (-14.4261, -19.241) -> (-14.4261, -19.4809) construction
  line L1011 (-14.4261, -19.4809) -> (-14.4261, -21.6323)
  spline S232 degree 2 poles (-14.4261, -21.6323) (-14.4261, -21.8283) (-14.1462, -22.1122) (-13.9502, -22.1122) knots 0 0 0 1 2 2 2
  line L1012 (-14.4261, -21.6323) -> (-14.4261, -21.8283) construction
  line L1013 (-14.4261, -21.8283) -> (-14.1462, -22.1122) construction
  line L1014 (-14.1462, -22.1122) -> (-13.9502, -22.1122) construction
  spline S233 degree 2 poles (-12.9945, -19.4809) (-12.9945, -19.241) (-12.7546, -19.241) knots 0 0 0 1 1 1
  line L1015 (-12.9945, -19.4809) -> (-12.9945, -19.241) construction
  line L1016 (-12.9945, -19.241) -> (-12.7546, -19.241) construction
  spline S234 degree 2 poles (-12.7546, -19.241) (-12.5146, -19.241) (-12.5146, -19.4809) knots 0 0 0 1 1 1
  line L1017 (-12.7546, -19.241) -> (-12.5146, -19.241) construction
  line L1018 (-12.5146, -19.241) -> (-12.5146, -19.4809) construction
  line L1019 (-12.5146, -19.4809) -> (-12.5146, -22.3521)
  spline S235 degree 2 poles (-12.5146, -22.3521) (-12.5146, -22.5921) (-12.7546, -22.5921) knots 0 0 0 1 1 1
  line L1020 (-12.5146, -22.3521) -> (-12.5146, -22.5921) construction
  line L1021 (-12.5146, -22.5921) -> (-12.7546, -22.5921) construction
  spline S236 degree 2 poles (-23.7635, -21.1565) (-24.0034, -21.1565) (-24.0034, -20.9165) knots 0 0 0 1 1 1
  line L1022 (-23.7635, -21.1565) -> (-24.0034, -21.1565) construction
  line L1023 (-24.0034, -21.1565) -> (-24.0034, -20.9165) construction
  spline S237 degree 2 poles (-24.0034, -20.9165) (-24.0034, -20.6766) (-23.7635, -20.6766) knots 0 0 0 1 1 1
  line L1024 (-24.0034, -20.9165) -> (-24.0034, -20.6766) construction
  line L1025 (-24.0034, -20.6766) -> (-23.7635, -20.6766) construction
  line L1026 (-23.7635, -20.6766) -> (-23.5235, -20.6766)
  spline S238 degree 2 poles (-23.5235, -20.6766) (-23.2996, -20.6766) (-23.1676, -20.5286) knots 0 0 0 1 1 1
  line L1027 (-23.5235, -20.6766) -> (-23.2996, -20.6766) construction
  line L1028 (-23.2996, -20.6766) -> (-23.1676, -20.5286) construction
  spline S239 degree 2 poles (-23.1676, -20.5286) (-23.0477, -20.3927) (-23.0477, -20.1967) knots 0 0 0 1 1 1
  line L1029 (-23.1676, -20.5286) -> (-23.0477, -20.3927) construction
  line L1030 (-23.0477, -20.3927) -> (-23.0477, -20.1967) construction
  spline S240 degree 2 poles (-23.0477, -20.1967) (-23.0477, -20.0008) (-23.1676, -19.8688) knots 0 0 0 1 1 1
  line L1031 (-23.0477, -20.1967) -> (-23.0477, -20.0008) construction
  line L1032 (-23.0477, -20.0008) -> (-23.1676, -19.8688) construction
  spline S241 degree 2 poles (-23.1676, -19.8688) (-23.2996, -19.7209) (-23.5275, -19.7209) knots 0 0 0 1 1 1
  line L1033 (-23.1676, -19.8688) -> (-23.2996, -19.7209) construction
  line L1034 (-23.2996, -19.7209) -> (-23.5275, -19.7209) construction
  line L1035 (-23.5275, -19.7209) -> (-23.7675, -19.7209)
  spline S242 degree 2 poles (-23.7675, -19.7209) (-24.0914, -19.7209) (-24.3393, -19.9128) knots 0 0 0 1 1 1
  line L1036 (-23.7675, -19.7209) -> (-24.0914, -19.7209) construction
  line L1037 (-24.0914, -19.7209) -> (-24.3393, -19.9128) construction
  spline S243 degree 2 poles (-24.3393, -19.9128) (-24.4113, -19.9648) (-24.4873, -19.9648) knots 0 0 0 1 1 1
  line L1038 (-24.3393, -19.9128) -> (-24.4113, -19.9648) construction
  line L1039 (-24.4113, -19.9648) -> (-24.4873, -19.9648) construction
  spline S244 degree 2 poles (-24.4873, -19.9648) (-24.5832, -19.9648) (-24.7272, -19.8168) (-24.7272, -19.7169) knots 0 0 0 1 2 2 2
  line L1040 (-24.4873, -19.9648) -> (-24.5832, -19.9648) construction
  line L1041 (-24.5832, -19.9648) -> (-24.7272, -19.8168) construction
  line L1042 (-24.7272, -19.8168) -> (-24.7272, -19.7169) construction
  spline S245 degree 2 poles (-24.7272, -19.7169) (-24.7272, -19.6049) (-24.6272, -19.5289) knots 0 0 0 1 1 1
  line L1043 (-24.7272, -19.7169) -> (-24.7272, -19.6049) construction
  line L1044 (-24.7272, -19.6049) -> (-24.6272, -19.5289) construction
  spline S246 degree 2 poles (-24.6272, -19.5289) (-24.2553, -19.241) (-23.7675, -19.241) knots 0 0 0 1 1 1
  line L1045 (-24.6272, -19.5289) -> (-24.2553, -19.241) construction
  line L1046 (-24.2553, -19.241) -> (-23.7675, -19.241) construction
  line L1047 (-23.7675, -19.241) -> (-23.5275, -19.241)
  spline S247 degree 2 poles (-23.5275, -19.241) (-23.0757, -19.241) (-22.8077, -19.5369) knots 0 0 0 1 1 1
  line L1048 (-23.5275, -19.241) -> (-23.0757, -19.241) construction
  line L1049 (-23.0757, -19.241) -> (-22.8077, -19.5369) construction
  spline S248 degree 2 poles (-22.8077, -19.5369) (-22.5678, -19.8088) (-22.5678, -20.1967) knots 0 0 0 1 1 1
  line L1050 (-22.8077, -19.5369) -> (-22.5678, -19.8088) construction
  line L1051 (-22.5678, -19.8088) -> (-22.5678, -20.1967) construction
  spline S249 degree 2 poles (-22.5678, -20.1967) (-22.5678, -20.6406) (-22.8677, -20.9165) knots 0 0 0 1 1 1
  line L1052 (-22.5678, -20.1967) -> (-22.5678, -20.6406) construction
  line L1053 (-22.5678, -20.6406) -> (-22.8677, -20.9165) construction
  spline S250 degree 2 poles (-22.8677, -20.9165) (-22.5678, -21.1925) (-22.5678, -21.6363) knots 0 0 0 1 1 1
  line L1054 (-22.8677, -20.9165) -> (-22.5678, -21.1925) construction
  line L1055 (-22.5678, -21.1925) -> (-22.5678, -21.6363) construction
  spline S251 degree 2 poles (-22.5678, -21.6363) (-22.5678, -22.0282) (-22.8077, -22.2961) knots 0 0 0 1 1 1
  line L1056 (-22.5678, -21.6363) -> (-22.5678, -22.0282) construction